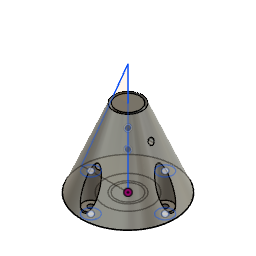
rod_connector v8 (Autodesk Fusion 360 design; units mm, degrees)
Autodesk Fusion 360 part; units mm, degrees
sketch "Sketch1" plane through (0, 0, 0) normal (0, 1, 0) x (1, 0, 0)
  circle A0 centre (0, 0) radius 6.4
  circle A1 centre (0, 0) radius 7.6
  circle A2 centre (0, 0) radius 12.5
  circle A3 centre (0, 0) radius 25
  circle A4 centre (-20, 0) radius 1.5
  circle A5 centre (0, -20) radius 1.5
  circle A6 centre (20, 0) radius 1.5
  circle A7 centre (0, 20) radius 1.5
  circle A8 centre (-20, 0) radius 4
  circle A9 centre (0, -20) radius 4
  circle A10 centre (20, 0) radius 4
  circle A11 centre (0, 20) radius 4
  dimension "d1" = 12.8
  dimension "d2" = 15.2
  dimension "d3" = 25
  dimension "d4" = 50
  dimension "d9" = 3
  dimension "d10" = 20
  dimension "d12" = 360
  dimension "d48" = 8
  dimension "d49" = 8
  dimension "d50" = 8
  dimension "d64" = 8
  measures "d1" diameter of A0
  measures "d2" diameter of A1
  measures "d3" diameter of A2
  measures "d4" diameter of A3
  measures "d9" diameter of A4
  measures "d10" distance of A0.centre A4.centre
  measures "d48" diameter of A8
  measures "d49" diameter of A9
  measures "d50" diameter of A10
  measures "d64" diameter of A11
sketch "Sketch3" plane through (0, 0, 0) normal (0, 0, 1) x (1, 0, 0)
  line L0 (0, 0) -> (0, 20)
  circle A0 centre (0, 20) radius 1.5
  dimension "d23" = 20
  dimension "d24" = 3
  measures "d23" distance of L0.start L0.end
  measures "d24" diameter of A0
sketch "Sketch5" plane through (0, 0, 0) normal (1, 0, 0) x (0, 0, -1)
  line L0 (0, 0) -> (0, 30)
  circle A0 centre (0, 30) radius 1.5
  dimension "d27" = 30
  dimension "d28" = 3
  measures "d27" distance of L0.start L0.end
  measures "d28" diameter of A0
sketch "Sketch6" plane through (0, 0, 0) normal (0, 0, 1) x (1, 0, 0)
  line L0 (0, 0) -> (-25, 0)
  line L1 (0, 0) -> (0, 60)
  line L2 (0, 60) -> (-25, 0)
  dimension "d38" = 25
  dimension "d71" = 60
  measures "d38" distance of L0.start L0.end
  measures "d71" distance of L0.start L1.end
revolve "Revolve2" add sketch "Sketch6" angle 360 about axis through (0, 0, 0) along (0, 1, 0)
extrude "Extrude16" cut sketch "Sketch1" along normal blind 70 contours A0 | A1
extrude "Extrude17" cut sketch "Sketch1" against normal blind 10 contours A0 | A1
extrude "Extrude18" add sketch "Sketch1" along normal blind 8 contours A1
extrude "Extrude19" add sketch "Sketch1" along normal blind 41.7 contours A0
extrude "Extrude20" cut sketch "Sketch1" along normal blind 20 contours A4 | A5 | A6 | A7
extrude "Extrude21" cut sketch "Sketch1" against normal blind 10 contours A4 | A5 | A6 | A7
extrude "Extrude22" cut sketch "Sketch1" along normal blind 30 contours A8 | A9 | A10 | A11
extrude "Extrude23" cut sketch "Sketch1" against normal blind 5 contours A8 | A9 | A10 | A11
extrude "Extrude24" add sketch "Sketch1" along normal blind 3.5 contours A8 | A9 | A10 | A11
extrude "Extrude25" cut sketch "Sketch3" along normal blind 20
extrude "Extrude26" cut sketch "Sketch3" against normal blind 20
extrude "Extrude27" cut sketch "Sketch5" along normal blind 20
extrude "Extrude28" cut sketch "Sketch5" against normal blind 20
